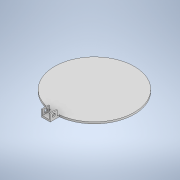
# Autodesk Inventor part: Tapacontenedor
Saved by Autodesk Inventor 2020.2 (Build 242310000, 310)
## iProperties
Created: 2020-10-22
Part Number: Tapacontenedor
Material: Generic
Document SubType Name: Modeling
Designer: JK
Density: 1 g/cm^3
Appearance: Default
Author: JK
Autodesk Inventor part; units mm, degrees
ref_plane "YZ Plane" through (0, 0, 0) normal (1, 0, 0) x (0, 1, 0)
ref_plane "XZ Plane" through (0, 0, 0) normal (0, 1, 0) x (-1, 0, 0)
ref_plane "XY Plane" through (0, 0, 0) normal (0, 0, 1) x (1, 0, 0)
sketch "Sketch1" plane through (0, 0, 0) normal (0, 1, 0) x (-1, 0, 0)
  circle A0 centre (0, 0) radius 45
  dimension "d0" = 90
  constraints: 1 centre point, 1 coincident
  measures "d0" diameter of A0
extrude "Extrusion1" add sketch "Sketch1" along normal blind 2
sketch "Sketch3" plane through (0, 0, 0) normal (1, 0, 0) x (0, 1, 0)
  line L0 (2, -45) -> (2, 45) projected
  line L1 (0, 15) -> (2, 15)
  line L2 (2, 15) -> (2, 55)
  line L3 (2, 55) -> (0, 55)
  line L4 (0, 55) -> (0, 15)
  line L5 (2, 55) -> (7.7736, 55)
  line L6 (7.7736, 55) -> (7.7736, 47)
  line L7 (7.7736, 47) -> (2, 47)
  line L8 (2, 47) -> (2, 55)
  point P0 (0, 0)
  point P1 (2, 15)
  point P2 (2, 47)
  dimension "d5" = 8
  dimension "d6" = 40
  dimension "d7" = 15
  constraints: 16 end point, 4 parallel, 2 horizontal, 2 perpendicular, 1 point on line
  measures "d5" distance of L5.end L6.end
  measures "d6" distance of L3.end L1.start
  measures "d7" distance from line of point (0, 0) L1
extrude "Extrusion2" add sketch "Sketch3" along normal mid plane 10
sketch "Sketch4" plane through (-5, 7.7736, 55) normal (0, 1, 0) x (1, 0, 0)
  line L0 (1.2, -4.8224) -> (8.8, -4.8224)
  line L1 (8.8, -4.8224) -> (8.8, 13.6038)
  line L2 (8.8, 13.6038) -> (1.2, 13.6038)
  line L3 (1.2, 13.6038) -> (1.2, -4.8224)
  line L4 (0, 0) -> (0, 8) projected
  line L5 (10, 8) -> (10, 0) projected
  point P0 (5, 55)
  dimension "d10" = 1.2
  dimension "d11" = 1.2
  constraints: 8 end point, 2 parallel, 1 horizontal, 1 perpendicular
  measures "d10" distance between parallel lines of L4 L3
  measures "d11" distance between parallel lines of L5 L1
extrude "Extrusion3" cut sketch "Sketch4" against normal up to surface (5.7736 mm away)
sketch "Sketch5" plane through (5, 0, 0) normal (1, 0, 0) x (0, 0, -1)
  circle A0 centre (-51, 4.7736) radius 1.85
  line L0 (-47, 2) -> (-47, 7.7736) projected
  line L1 (-47, 7.7736) -> (-55, 7.7736) projected
  point P0 (0, 0)
  dimension "d14" = 3.7
  dimension "d15" = 4
  dimension "d16" = 3
  constraints: 1 centre point
  measures "d14" diameter of A0
  measures "d15" distance from line of L0 A0.centre
  measures "d16" distance from line of L1 A0.centre
extrude "Extrusion4" cut sketch "Sketch5" against normal blind 13
body "Solid1"
